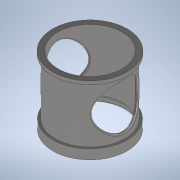
# Autodesk Inventor part: Стакан1
Saved by Autodesk Inventor 2021 (Build 250183000, 183)
## iProperties
Created: 2020-11-15
Part Number: Стакан1
Material: Сталь, высокопрочная, низколегированная
Document SubType Name: Modeling
Designer: Тимоха
Density: 7.85 g/cm^3
Appearance: Сталь — полированная
Mass: 2535.61 g
Surface Area: 1130.45 cm^2
Volume: 323.008 cm^3
Author: Тимоха
Autodesk Inventor part; units mm, degrees
ref_plane "YZ Plane" through (0, 0, 0) normal (1, 0, 0) x (0, 1, 0)
ref_plane "XZ Plane" through (0, 0, 0) normal (0, 1, 0) x (-1, 0, 0)
ref_plane "XY Plane" through (0, 0, 0) normal (0, 0, 1) x (1, 0, 0)
sketch "Эскиз1" plane through (0, 0, 0) normal (0, 0, 1) x (1, 0, 0)
  line L0 (0, 0) -> (70, 0)
  line L1 (70, 0) -> (78, 0)
  line L2 (0, 0) -> (0, 150)
  line L3 (78, 0) -> (78, 20)
  line L4 (78, 20) -> (73, 20)
  line L5 (73, 20) -> (73, 137)
  line L6 (67, 144) -> (67, 15.8104)
  line L7 (67, 15.8104) -> (72, 10)
  line L8 (72, 10) -> (72, 0)
  line L9 (73, 137) -> (78.5, 137)
  line L10 (78.5, 137) -> (78.5, 144)
  line L11 (78.5, 144) -> (67, 144)
  point P0 (67.5, 0)
  dimension "d2" = 150
  dimension "d3" = 20
  dimension "d4" = 5
  dimension "d5" = 117
  dimension "d14" = 5.5
  dimension "d16" = 124
  dimension "d17" = 72
  dimension "d18" = 6
  constraints: 24 end point, 4 perpendicular, 3 vertical, 2 horizontal, 2 point on line, 1 parallel
  measures "d2" distance of L0.start L2.end
  measures "d3" distance of L1.end L3.end
  measures "d4" distance of L3.end L4.end
  measures "d5" distance of L4.end L5.end
  measures "d14" distance of L5.end L9.end
  measures "d16" distance between parallel lines of L11 L4
  measures "d17" distance of L8.end L0.start
  measures "d18" distance of L1.end L8.end
revolve "Вращение1" add sketch "Эскиз1" angle 360 about axis through (0, 0, 0) along (0, 1, 0)
sketch "Эскиз2" plane through (0, 0, 0) normal (1, 0, 0) x (0, 1, 0)
  line L0 (0, 0) -> (79, 0)
  circle A0 centre (79, 0) radius 47.5
  dimension "d9" = 79
  dimension "d10" = 95
  constraints: 2 end point, 1 centre point, 1 coincident, 1 horizontal
  measures "d9" distance of L0.start L0.end
  measures "d10" diameter of A0
extrude "Выдавливание1" cut sketch "Эскиз2" along normal through all both and the other way through all
fillet "Сопряжение1" radius 2.5 6 edges at (-73, 31.5, -0.003) (-67, 31.5, -0.0055) (55.4324, 79.0009, -47.5) (55.4324, 78.9991, 47.5) (47.252, 78.9985, 47.5) (47.252, 79.0015, -47.5)
chamfer "Фаска1" distance 2 angle 45 1 edges at (-72, 0, 0)
